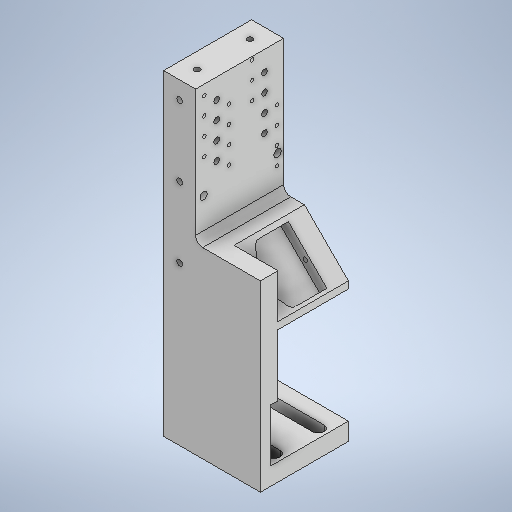
# Autodesk Inventor part: 1inchTurningPeriscope
Saved by Autodesk Inventor 2025 (Build 290162010, 162A)
## iProperties
Created: 2025-07-15
Part Number: 1inchTurningPeriscope
Material: Generic
Document SubType Name: Modeling
Designer: luttmann
Density: 1 g/cm^3
Appearance: Default
Author: luttmann
Autodesk Inventor part; units mm, degrees
ref_plane "YZ Plane" through (0, 0, 0) normal (1, 0, 0) x (0, 1, 0)
ref_plane "XZ Plane" through (0, 0, 0) normal (0, 1, 0) x (-1, 0, 0)
ref_plane "XY Plane" through (0, 0, 0) normal (0, 0, 1) x (1, 0, 0)
sketch "Sketch1" plane through (0, 0, 0) normal (0, 1, 0) x (-1, 0, 0)
  line L0 (23.4974, 39.0825) -> (-51.5026, 39.0825)
  line L1 (-51.5026, 39.0825) -> (-51.5026, -35.9175)
  line L2 (-51.5026, -35.9175) -> (23.4974, -35.9175)
  line L3 (23.4974, -35.9175) -> (23.4974, 39.0825)
  point P0 (0, 0)
  dimension "d0" = 75
  dimension "d1" = 75
  constraints: 8 end point, 2 parallel, 1 horizontal, 1 perpendicular
  measures "d0" distance of L2.end L0.start
  measures "d1" distance of L0.start L0.end
extrude "Extrusion1" add sketch "Sketch1" along normal blind 10
sketch "Sketch2" plane through (0, 10, 0) normal (0, 1, 0) x (1, 0, 0)
  line L0 (-23.4974, 35.9175) -> (-23.4974, -39.0825) projected
  line L1 (51.5026, -39.0825) -> (51.5026, 35.9175) projected
  line L2 (-23.4974, -39.0825) -> (51.5026, -39.0825)
  line L3 (51.5026, -39.0825) -> (51.5026, -29.0825)
  line L4 (51.5026, -29.0825) -> (-23.4974, -29.0825)
  line L5 (-23.4974, -29.0825) -> (-23.4974, -39.0825)
  point P0 (0, 0)
  point P1 (-23.4974, -29.0825)
  dimension "d4" = 10
  constraints: 8 end point, 2 parallel, 1 horizontal, 1 perpendicular, 1 point on line
  measures "d4" distance between parallel lines of L2 L4
extrude "Extrusion2" add sketch "Sketch2" along normal blind 100
sketch "Sketch3" plane through (0, 10, 0) normal (0, 1, 0) x (1, 0, 0)
  line L0 (51.5026, 35.9175) -> (-23.4974, 35.9175) projected
  line L1 (51.5026, -29.0825) -> (-23.4974, -29.0825) projected
  line L2 (-23.4974, 35.9175) -> (-13.4974, 35.9175)
  line L3 (-13.4974, 35.9175) -> (-13.4974, -29.0825)
  line L4 (-13.4974, -29.0825) -> (-23.4974, -29.0825)
  line L5 (-23.4974, -29.0825) -> (-23.4974, 35.9175)
  point P0 (0, 0)
  dimension "d7" = 10
  constraints: 8 end point, 2 parallel, 1 horizontal, 1 perpendicular, 1 point on line
  measures "d7" distance between parallel lines of L3 L5
extrude "Extrusion3" add sketch "Sketch3" along normal blind 200
sketch "Sketch8" plane through (-13.4974, 10, 29.0825) normal (1, 0, 0) x (0, 0, -1)
  line L0 (-10, -10) -> (-10, 100) projected
  line L1 (65, -10) -> (65, 200) projected
  line L2 (-10, 100) -> (65, 100)
  line L3 (65, 100) -> (65, 170)
  line L4 (65, 170) -> (-10, 170)
  line L5 (-10, 170) -> (-10, 100)
  line L6 (-10, 100) -> (0, 100) projected
  point P0 (29.0825, -10)
  dimension "d26" = 0
  dimension "d27" = 70
  constraints: 8 end point, 2 parallel, 2 point on line, 1 horizontal, 1 perpendicular
  measures "d26" distance between parallel lines of L6 L2
  measures "d27" distance of L4.end L2.start
extrude "Extrusion5" add sketch "Sketch8" along normal blind 8.2 and the other way blind 10
sketch "Sketch9" plane through (-5.2974, 10, 29.0825) normal (1, 0, 0) x (0, 0, -1)
  line L0 (-10, -10) -> (65, -10) projected
  line L1 (-10, -10) -> (-10, 100) projected
  point P0 (29.0825, -10)
  point P1 (1.922, 128.721)
  dimension "d32" = 138.721
  dimension "d33" = 11.922
  measures "d32" distance from line of L0 point (1.922, 128.721)
  measures "d33" distance from line of L1 point (1.922, 128.721)
hole "Hole2" at (-5.2974, 138.721, 27.1605) direction (-1, 0, 0) diameter 3.242 end through all thread size "M4x0.7" class "6H" standard "ANSI Metric M Profile"
sketch "Sketch10" plane through (-23.4974, 0, -35.9175) normal (-1, 0, 0) x (0, 0, 1)
  line L0 (0, 210) -> (65, 210) projected
  line L1 (0, 0) -> (15, 0)
  line L2 (15, 0) -> (15, 210)
  line L3 (15, 210) -> (0, 210)
  line L4 (0, 210) -> (0, 0)
  point P0 (35.9175, 0)
  dimension "d41" = 15
  constraints: 8 end point, 2 parallel, 1 horizontal, 1 perpendicular, 1 point on line
  measures "d41" distance between parallel lines of L2 L4
extrude "Extrusion6" cut sketch "Sketch10" against normal blind 77.4125
sketch "Sketch12" plane through (-5.2974, 10, 29.0825) normal (1, 0, 0) x (0, 0, -1)
  circle A0 centre (1.922, 128.721) radius 1.621 projected
  point P0 (29.0825, -10)
  point P1 (29.122, 128.721)
  dimension "d65" = 27.2
  measures "d65" distance of A0.centre point (29.122, 128.721)
hole "Hole5" at (-5.2974, 138.721, -0.0395) direction (-1, 0, 0) diameter 3.242 end through all thread size "M4x0.7" class "6H" standard "ANSI Metric M Profile"
sketch "Sketch18" plane through (51.5026, 0, 39.0825) normal (1, 0, 0) x (0, 0, -1)
  line L0 (60, 210) -> (60, 0) projected
  line L1 (60, 0) -> (50, 0)
  line L2 (50, 0) -> (50, 180)
  line L3 (50, 180) -> (60, 180)
  line L4 (60, 180) -> (60, 0)
  point P0 (60, 130)
  point P1 (60, 180)
  dimension "d118" = 10
  constraints: 8 end point, 2 parallel, 1 horizontal, 1 perpendicular
  measures "d118" distance between parallel lines of L4 L2
extrude "Extrusion10" cut sketch "Sketch18" against normal blind 83.6625
sketch "Sketch19" plane through (51.5026, 0, -10.9175) normal (0, 0, -1) x (-1, 0, 0)
  line L0 (75, 0) -> (0, 0) projected
  line L1 (0, 0) -> (20, 0)
  line L2 (20, 0) -> (20, 136.0118)
  line L3 (20, 136.0118) -> (0, 136.0118)
  line L4 (0, 136.0118) -> (0, 0)
  point P0 (51.5026, 0)
  point P1 (20, 0)
  dimension "d121" = 20
  constraints: 8 end point, 2 parallel, 1 horizontal, 1 perpendicular
  measures "d121" distance of L2.end L3.end
extrude "Extrusion11" cut sketch "Sketch19" against normal blind 53.7125
sketch "Sketch20" plane through (-5.2974, 110, 29.0825) normal (0, 0, -1) x (-1, 0, 0)
  line L0 (-36.8, -31) -> (8.2, 14)
  line L1 (8.2, 14) -> (8.2, -31)
  line L2 (8.2, -31) -> (-36.8, -31)
  line L3 (8.2, 14) -> (8.2, -31)
  line L4 (18.2, -110) -> (-36.8, -110) projected
  point P0 (-5.2974, -110)
  dimension "d124" = 45
  dimension "d125" = 79
  constraints: 8 end point, 2 perpendicular, 1 vertical
  measures "d124" angle of L2 L0
  measures "d125" distance between parallel lines of L4 L2
extrude "Extrusion12" add sketch "Sketch20" along normal blind 40
sketch "Sketch22" plane through (-3.8064, 114.309, -10.9175) normal (0.7071068, 0.7071068, 0) x (-0.7071068, 0.7071068, 0)
  circle A0 centre (-33.8125, 24.6) radius 12.7
  line L0 (-49.9345, 40) -> (-49.9345, 0) projected
  point P0 (-83.5202, 10.9175)
  dimension "d129" = 25.4
  dimension "d130" = 16.122
  constraints: 1 centre point
  measures "d129" diameter of A0
  measures "d130" distance from line of L0 A0.centre
sketch "Sketch23" plane through (-13.4974, 79, 29.0825) normal (0, -1, 0) x (1, 0, 0)
  line L0 (45, 0) -> (45, -40) projected
  line L1 (0, 0) -> (45, 0) projected
  line L2 (45, -40) -> (0, -40)
  line L3 (0, -40) -> (0, 0)
  line L4 (0, 0) -> (45, 0)
  line L5 (45, 0) -> (45, -40)
  point P0 (13.4974, -29.0825)
  constraints: 8 end point, 2 parallel, 1 horizontal, 1 perpendicular
extrude "Extrusion13" add sketch "Sketch23" along normal blind 4
extrude "Extrusion14" cut sketch "Sketch22" against normal blind 6
sketch "Sketch24" plane through (-5.2974, 110, 29.0825) normal (0, 0, 1) x (1, 0, 0)
  line L0 (0, 5.8) -> (36.8, -31) projected
  line L1 (0, 0) -> (36.8, 0) projected
  line L2 (0, 5.8) -> (0, 0)
  line L3 (0, 0) -> (6.0337, 0)
  line L4 (6.0337, 0) -> (0, 5.8)
  point P0 (5.2974, -110)
  point P1 (5.8, 0)
  constraints: 6 end point, 1 point on line, 1 vertical
extrude "Extrusion15" cut sketch "Sketch24" against normal blind 47.975 contours L0 L1 L2
sketch "Sketch27" plane through (0, 110, 0) normal (0, 1, 0) x (1, 0, 0)
  line L0 (-23.4974, -39.0825) -> (31.5026, -39.0825) projected
  line L1 (-13.4974, -29.0825) -> (31.5026, -29.0825) projected
  line L2 (31.5026, -39.0825) -> (31.5026, -29.0825)
  line L3 (31.5026, -29.0825) -> (6.5026, -29.0825)
  line L4 (6.5026, -29.0825) -> (6.5026, 10.9175)
  line L5 (31.5026, 10.9175) -> (-13.4974, 10.9175) projected
  line L6 (-5.2974, -39.0825) -> (-5.2974, 10.9175) projected
  line L7 (6.5026, 10.9175) -> (-5.2974, 10.9175)
  line L8 (-5.2974, 10.9175) -> (-5.2974, -39.0825)
  line L9 (-5.2974, -39.0825) -> (31.5026, -39.0825)
  line L10 (31.5026, -29.0825) -> (31.5026, 10.9175) projected
  point P0 (0, 0)
  dimension "d138" = 25
  constraints: 12 end point, 4 perpendicular, 2 point on line, 1 parallel, 1 vertical
  measures "d138" distance between parallel lines of L2 L4
extrude "Extrusion16" cut sketch "Sketch27" against normal blind 6 contours L6 L1 L2 L0 | L6 L5 L4 L1
sketch "Sketch28" plane through (-13.4974, 180, -10.9175) normal (0, 0, -1) x (-1, 0, 0)
  line L0 (-20, -76) -> (-45, -101) projected
  line L1 (-45, -105) -> (-45, -170) projected
  point P0 (-13.4974, -180)
  point P1 (-31.4787, -91.7213)
  dimension "d142" = 3
  dimension "d143" = 13.5213
  measures "d142" distance from line of L0 point (-31.479, -91.721)
  measures "d143" distance from line of L1 point (-31.479, -91.721)
hole "Hole8" at (17.9812, 88.2787, -10.9175) direction (0, 0, 1) diameter 2.459 depth 13 tip angle 118 thread size "M3x0.5" class "6H" standard "ANSI Metric M Profile"
sketch "Sketch29" plane through (31.5026, 79, -10.9175) normal (0.7071068, 0.7071068, 0) x (-0.7071068, 0.7071068, 0)
  line L0 (16, 39.147) -> (32.7002, 30)
  line L1 (32.7002, 30) -> (32.7002, 11)
  line L2 (32.7002, 11) -> (1.7002, 11)
  line L3 (1.7002, 11) -> (1.7002, 31)
  line L4 (1.7002, 31) -> (16, 39.147)
  circle A0 centre (16.122, 24.6) radius 12.7 projected
  line L5 (0, 40) -> (0, 0) projected
  line L6 (35.3553, 0) -> (0, 0) projected
  point P0 (-33.5858, 10.9175)
  dimension "d151" = 16
  dimension "d152" = 19
  dimension "d153" = 20
  dimension "d154" = 31
  dimension "d300" = 11
  constraints: 10 end point, 2 perpendicular, 2 tangent, 1 vertical
  measures "d151" distance from line of L5 L0.start
  measures "d152" distance of L0.end L1.end
  measures "d153" distance of L2.end L3.end
  measures "d154" distance of L1.end L2.end
  measures "d300" distance between parallel lines of L6 L2
extrude "Extrusion17" cut sketch "Sketch29" against normal blind 6
sketch "Sketch30" plane through (-13.4974, 180, 29.0825) normal (1, 0, 0) x (0, 0, -1)
  line L0 (0, 0) -> (0, 30) projected
  line L1 (50, 30) -> (50, 0) projected
  line L2 (0, 30) -> (50, 30)
  line L3 (50, 30) -> (50, 0)
  line L4 (50, 0) -> (0, 0)
  line L5 (0, 0) -> (0, 30)
  point P0 (29.0825, -180)
  constraints: 8 end point, 2 parallel, 1 horizontal, 1 perpendicular
extrude "Extrusion18" cut sketch "Sketch30" against normal through all
sketch "Sketch31" plane through (-5.2974, 10, 29.0825) normal (1, 0, 0) x (0, 0, -1)
  circle A0 centre (1.922, 128.721) radius 1.621 projected
  circle A1 centre (29.122, 128.721) radius 1.621 projected
  point P0 (29.0825, -10)
  point P1 (1.922, 138.721)
  point P2 (29.122, 138.721)
  point P3 (1.922, 148.721)
  point P4 (29.122, 148.721)
  point P5 (1.922, 158.721)
  point P6 (29.122, 158.721)
  dimension "d160" = 10
  dimension "d161" = 10
  dimension "d162" = 10
  dimension "d163" = 10
  dimension "d164" = 27.2
  dimension "d165" = 27.2
  dimension "d166" = 10
  dimension "d167" = 10
  dimension "d168" = 27.2
  measures "d160" distance of A0.centre point (1.922, 138.721)
  measures "d161" distance of point (1.922, 148.721) point (1.922, 138.721)
  measures "d162" distance of A1.centre point (29.122, 138.721)
  measures "d163" distance of point (29.122, 148.721) point (29.122, 138.721)
  measures "d164" distance of point (29.122, 138.721) point (1.922, 138.721)
  measures "d165" distance of point (29.122, 148.721) point (1.922, 148.721)
  measures "d166" distance of point (1.922, 158.721) point (1.922, 148.721)
  measures "d167" distance of point (29.122, 148.721) point (29.122, 158.721)
  measures "d168" distance of point (1.922, 158.721) point (29.122, 158.721)
hole "Hole9" at (-5.2974, 148.721, 27.1605) at (-5.2974, 148.721, -0.0395) at (-5.2974, 158.721, 27.1605) at (-5.2974, 158.721, -0.0395) at (-5.2974, 168.721, 27.1605) at (-5.2974, 168.721, -0.0395) direction (-1, 0, 0) diameter 3.242 end through all thread size "M4x0.7" class "6H" standard "ANSI Metric M Profile"
sketch "Sketch32" plane through (-5.2974, 10, 29.0825) normal (1, 0, 0) x (0, 0, -1)
  line L0 (-9.8792, 104.3333) -> (24.1779, 138.3904)
  line L1 (-10, 94) -> (-10, 170) projected
  circle A0 centre (1.922, 128.721) radius 1.621 projected
  line L2 (5.5557, 144.9412) -> (-21.8511, 117.5344)
  line L3 (3.165, 152.5505) -> (-26.8557, 122.5298)
  line L4 (23.7288, 147.9413) -> (-8.7448, 115.4677)
  circle A1 centre (1.922, 138.721) radius 1.621 projected
  line L5 (23.2486, 157.4611) -> (-6.4533, 127.7592)
  line L6 (6.1423, 165.5278) -> (-25.5427, 133.8428)
  circle A2 centre (1.922, 148.721) radius 1.621 projected
  line L7 (18.2486, 162.4611) -> (-6.1016, 138.1109)
  line L8 (8.2366, 177.6221) -> (-21.709, 147.6765)
  circle A3 centre (1.922, 158.721) radius 1.621 projected
  line L9 (-5.078, 175.088) -> (-5.078, 99.3059)
  line L10 (8.922, 175.0874) -> (8.922, 95.9878)
  point P0 (29.0825, -10)
  point P1 (-5.078, 134.3075)
  point P2 (-5.078, 144.3075)
  point P3 (-5.078, 154.3075)
  point P4 (-5.078, 164.3075)
  point P5 (8.922, 153.1345)
  point P6 (8.922, 143.1345)
  point P7 (8.922, 133.1345)
  point P8 (8.922, 123.1345)
  dimension "d176" = -45
  dimension "d177" = 8.9
  dimension "d178" = 8.9
  dimension "d179" = 8.9
  dimension "d180" = 8.9
  dimension "d181" = 8.9
  dimension "d182" = 8.9
  dimension "d183" = 8.9
  dimension "d184" = 8.9
  dimension "d185" = 7
  dimension "d186" = 7
  constraints: 20 end point, 16 point on line, 9 parallel, 1 vertical
  measures "d176" angle of L1 L0
  measures "d177" distance from line of L0 A0.centre
  measures "d178" distance from line of L2 A0.centre
  measures "d179" distance from line of L3 A1.centre
  measures "d180" distance from line of A1.centre L4
  measures "d181" distance from line of A2.centre L5
  measures "d182" distance from line of L6 A2.centre
  measures "d183" distance from line of A3.centre L7
  measures "d184" distance from line of A3.centre L8
  measures "d185" distance from line of L9 A3.centre
  measures "d186" distance from line of A3.centre L10
hole "Hole10" at (-5.2974, 144.3075, 34.1605) at (-5.2974, 154.3075, 34.1605) at (-5.2974, 164.3075, 34.1605) at (-5.2974, 174.3075, 34.1605) at (-5.2974, 163.1345, 20.1605) at (-5.2974, 153.1345, 20.1605) at (-5.2974, 143.1345, 20.1605) at (-5.2974, 133.1345, 20.1605) direction (-1, 0, 0) diameter 2 depth 5
sketch "Sketch33" plane through (-5.2974, 10, 29.0825) normal (1, 0, 0) x (0, 0, -1)
  line L0 (53.8181, 116.6114) -> (12.0431, 158.3864)
  line L1 (32.543, 112.7135) -> (-4.6883, 149.9448)
  line L2 (40, 94) -> (40, 170) projected
  circle A0 centre (29.122, 128.721) radius 1.621 projected
  line L3 (54.3802, 126.0493) -> (18.9851, 161.4444)
  line L4 (36.6834, 118.5731) -> (-1.4226, 156.6791)
  circle A1 centre (29.122, 138.721) radius 1.621 projected
  line L5 (54.2793, 136.1502) -> (12.9965, 177.433)
  line L6 (38.6694, 126.5871) -> (8.0905, 157.166)
  circle A2 centre (29.122, 148.721) radius 1.621 projected
  line L7 (53.1504, 147.2791) -> (17.9965, 182.433)
  line L8 (42.6319, 132.6246) -> (17.9624, 157.2941)
  circle A3 centre (29.122, 158.721) radius 1.621 projected
  line L9 (22.122, 175.4576) -> (22.122, 100.5612)
  line L10 (36.122, 181.9966) -> (36.122, 101.1703)
  point P0 (29.0825, -10)
  point P1 (22.122, 148.3075)
  point P2 (22.122, 158.3075)
  point P3 (22.122, 168.3075)
  point P4 (22.122, 178.3075)
  point P5 (36.122, 129.1345)
  point P6 (36.122, 119.1345)
  point P7 (36.122, 109.1345)
  point P8 (36.122, 139.1345)
  dimension "d194" = -45
  dimension "d195" = 8.9
  dimension "d196" = 8.9
  dimension "d197" = 8.9
  dimension "d198" = 8.9
  dimension "d199" = 8.9
  dimension "d200" = 8.9
  dimension "d201" = 8.9
  dimension "d202" = 8.9
  dimension "d203" = 7
  dimension "d204" = 7
  constraints: 20 end point, 16 point on line, 9 parallel, 1 vertical
  measures "d194" angle of L2 L0
  measures "d195" distance from line of L0 A0.centre
  measures "d196" distance from line of A0.centre L1
  measures "d197" distance from line of L3 A1.centre
  measures "d198" distance from line of L4 A1.centre
  measures "d199" distance from line of A2.centre L5
  measures "d200" distance from line of L6 A2.centre
  measures "d201" distance from line of L7 A3.centre
  measures "d202" distance from line of L8 A3.centre
  measures "d203" distance from line of L9 A3.centre
  measures "d204" distance from line of A3.centre L10
hole "Hole12" at (-5.2974, 158.3075, 6.9605) at (-5.2974, 168.3075, 6.9605) at (-5.2974, 178.3075, 6.9605) at (-5.2974, 188.3075, 6.9605) at (-5.2974, 139.1345, -7.0395) at (-5.2974, 129.1345, -7.0395) at (-5.2974, 119.1345, -7.0395) at (-5.2974, 149.1345, -7.0395) direction (-1, 0, 0) diameter 2 depth 5
sketch "Sketch38" plane through (0, 10, 0) normal (0, 1, 0) x (1, 0, 0)
  line L0 (-8.0741, -13.6825) -> (25.852, -13.6825)
  line L1 (-23.4974, -39.0825) -> (31.5026, -39.0825) projected
  line L2 (-4.4974, -26.1825) -> (26.5026, -26.1825) construction
  line L3 (-23.4974, 10.9175) -> (-23.4974, -39.0825) projected
  line L4 (-4.4974, -29.4825) -> (26.5026, -29.4825)
  line L5 (26.5026, -22.8825) -> (-4.4974, -22.8825)
  arc A0 (-4.4974, -22.8825) -> (-4.4974, -29.4825) centre (-4.4974, -26.1825) ccw
  arc A1 (26.5026, -29.4825) -> (26.5026, -22.8825) centre (26.5026, -26.1825) ccw
  line L6 (31.5026, -29.0825) -> (31.5026, 10.9175) projected
  line L7 (-4.4974, -1.1825) -> (26.5026, -1.1825) construction
  line L8 (-4.4974, -4.4825) -> (26.5026, -4.4825)
  line L9 (26.5026, 2.1175) -> (-4.4974, 2.1175)
  arc A2 (-4.4974, 2.1175) -> (-4.4974, -4.4825) centre (-4.4974, -1.1825) ccw
  arc A3 (26.5026, -4.4825) -> (26.5026, 2.1175) centre (26.5026, -1.1825) ccw
  point P0 (0, 0)
  point P1 (11.0026, -26.1825)
  point P2 (11.0026, -1.1825)
  dimension "d236" = 25.4
  dimension "d237" = 12.5
  dimension "d238" = 3.3
  dimension "d239" = 31
  dimension "d240" = 5
  dimension "d241" = 31
  dimension "d242" = 5
  dimension "d243" = 3.3
  dimension "d244" = 12.5
  constraints: 18 end point, 8 point on circle, 8 tangent, 4 centre point, 2 horizontal, 2 midpoint, 2 parallel, 1 perpendicular
  measures "d236" distance between parallel lines of L1 L0
  measures "d237" distance from line of L0 L2.start
  measures "d238" radius of A0
  measures "d239" distance of L5.start L5.end
  measures "d240" distance from line of L6 L2.end
  measures "d241" distance of L9.start L9.end
  measures "d242" distance from line of L6 L7.end
  measures "d243" radius of A2
  measures "d244" distance from line of L0 L7.end
extrude "Extrusion22" cut sketch "Sketch38" against normal through all
fillet "Fillet2" radius 4 5 edges at (-13.4974, 75, 9.0825) (28.1783, 78.0802, 20.0825) (18.0668, 88.1917, 28.2295) (6.258, 100.0005, 19.0825) (-5.2974, 104, 14.0825)
sketch "Sketch40" plane through (-5.2974, 10, 29.0825) normal (1, 0, 0) x (0, 0, -1)
  line L0 (0, 0) -> (40, 0) projected
  line L1 (-10, 98) -> (-10, 170) projected
  circle A0 centre (29.122, 128.721) radius 1.621 projected
  point P0 (29.0825, -10)
  point P1 (-5.5, 115.243)
  point P2 (-5, 0)
  point P3 (36.544, 115.243)
  dimension "d252" = 115.243
  dimension "d253" = 4.5
  dimension "d254" = 7.422
  measures "d252" distance from line of L0 point (-5.5, 115.243)
  measures "d253" distance from line of L1 point (-5.5, 115.243)
  measures "d254" horizontal distance of A0.centre point (36.544, 115.243)
hole "Hole13" at (-5.2974, 125.243, 34.5825) at (-5.2974, 125.243, -7.4615) direction (-1, 0, 0) diameter 4.2 end through all clearance for "Flat Head Machine Screw" size "M4" standard "Ansi Metric M Profile"
sketch "Sketch41" plane through (-5.2974, 180, -10.9175) normal (0, 0, -1) x (-1, 0, 0)
  line L0 (18.2, 0) -> (18.2, -180) projected
  line L1 (18.2, -180) -> (-36.8, -180) projected
  point P0 (-5.2974, -180)
  point P1 (9.1, -90)
  point P2 (9.1, -50)
  point P3 (9.1, -10)
  dimension "d262" = 9.1
  dimension "d263" = 9.1
  dimension "d264" = 9.1
  dimension "d265" = 90
  dimension "d266" = 40
  dimension "d267" = 40
  measures "d262" distance from line of L0 point (9.1, -90)
  measures "d263" distance from line of L0 point (9.1, -50)
  measures "d264" distance from line of L0 point (9.1, -10)
  measures "d265" distance from line of L1 point (9.1, -90)
  measures "d266" distance of point (9.1, -90) point (9.1, -50)
  measures "d267" distance of point (9.1, -50) point (9.1, -10)
hole "Hole14" at (-14.3974, 90, -10.9175) at (-14.3974, 130, -10.9175) at (-14.3974, 170, -10.9175) direction (0, 0, 1) diameter 3.242 depth 7.8 thread size "M4x0.7" class "6H" standard "ANSI Metric M Profile"
sketch "Sketch42" plane through (-23.4974, 180, 39.0825) normal (0, 0, 1) x (1, 0, 0)
  circle A0 centre (9.1, -10) radius 1.621 projected
  circle A1 centre (9.1, -50) radius 1.621 projected
  line L0 (0, -180) -> (0, 0) projected
  line L1 (0, -180) -> (55, -180) projected
  point P0 (23.4974, -180)
  point P1 (9.1, -90)
  dimension "d275" = 9.1
  dimension "d276" = 9.1
  dimension "d277" = 9.1
  dimension "d278" = 90
  dimension "d279" = 40
  dimension "d280" = 40
  constraints: 2 coincident
  measures "d275" distance from line of L0 point (9.1, -90)
  measures "d276" distance from line of L0 A1.centre
  measures "d277" distance from line of L0 A0.centre
  measures "d278" distance from line of L1 point (9.1, -90)
  measures "d279" distance of point (9.1, -90) A1.centre
  measures "d280" distance of A1.centre A0.centre
hole "Hole15" at (-14.3974, 170, 39.0825) at (-14.3974, 130, 39.0825) at (-14.3974, 90, 39.0825) direction (0, 0, -1) diameter 3.242 depth 7.8 thread size "M4x0.7" class "6H" standard "ANSI Metric M Profile"
sketch "Sketch43" plane through (-23.4974, 180, 39.0825) normal (0, 1, 0) x (1, 0, 0)
  line L0 (0, 0) -> (0, 50) projected
  line L1 (0, 0) -> (18.2, 0) projected
  line L2 (18.2, 50) -> (0, 50) projected
  point P0 (23.4974, 39.0825)
  point P1 (9.1, 10)
  point P2 (9.1, 40)
  dimension "d288" = 9.1
  dimension "d289" = 9.1
  dimension "d290" = 10
  dimension "d291" = 10
  dimension "d292" = 30
  measures "d288" distance from line of L0 point (9.1, 10)
  measures "d289" distance from line of L0 point (9.1, 40)
  measures "d290" distance from line of L1 point (9.1, 10)
  measures "d291" distance from line of L2 point (9.1, 40)
  measures "d292" distance of point (9.1, 40) point (9.1, 10)
hole "Hole16" at (-14.3974, 180, 29.0825) at (-14.3974, 180, -0.9175) direction (0, -1, 0) diameter 3.242 depth 7.8 thread size "M4x0.7" class "6H" standard "ANSI Metric M Profile"
sketch "Sketch44" plane through (31.5026, 0, -10.9175) normal (1, 0, 0) x (0, 0, -1)
  line L0 (-40, 75) -> (-40, 10) projected
  line L1 (-40, 10) -> (-44, 10)
  line L2 (-44, 10) -> (-44, 40)
  line L3 (-44, 40) -> (-40, 40)
  line L4 (-40, 40) -> (-40, 10)
  point P0 (-10.9175, 0)
  point P1 (-40, 40)
  dimension "d301" = 30
  dimension "d302" = 4
  constraints: 8 end point, 2 parallel, 1 horizontal, 1 perpendicular
  measures "d301" distance of L1.end L2.end
  measures "d302" distance of L0.end L1.end
extrude "Extrusion24" cut sketch "Sketch44" against normal blind 45
fillet "Fillet3" radius 4 1 edges at (-13.4974, 10, 11.0825)
fillet "Fillet5" radius 4 1 edges at (-13.4974, 40, 31.0825)
equation "\"d65\" = d62"
equation "\"d161\" = d160"
equation "\"d162\" = d160"
equation "\"d163\" = d160"
equation "\"d166\" = d160"
equation "\"d167\" = d160"
equation "\"d178\" = d177"
equation "\"d179\" = d177"
equation "\"d180\" = d177"
equation "\"d181\" = d177"
equation "\"d182\" = d177"
equation "\"d183\" = d177"
equation "\"d184\" = d177"
equation "\"d195\" = d177"
equation "\"d196\" = d177"
equation "\"d197\" = d177"
equation "\"d198\" = d177"
equation "\"d199\" = d177"
equation "\"d200\" = d177"
equation "\"d201\" = d177"
equation "\"d202\" = d177"
equation "\"d263\" = d262"
equation "\"d264\" = d262"
equation "\"d62\" = 27.2"
body "Solid1"
